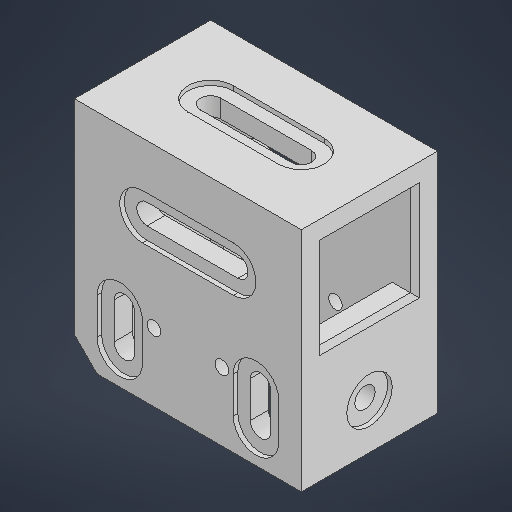
# Autodesk Inventor part: Part1
Saved by Autodesk Inventor 2025.1 (Build 291241000, 241)
## iProperties
Created: 2025-03-06
Part Number: Part1
Material: Generic
Document SubType Name: Modeling
Designer: jerem
Density: 1 g/cm^3
Appearance: Default
Author: jerem
Autodesk Inventor part; units mm, degrees
ref_plane "YZ Plane" through (0, 0, 0) normal (1, 0, 0) x (0, 1, 0)
ref_plane "XZ Plane" through (0, 0, 0) normal (0, 1, 0) x (-1, 0, 0)
ref_plane "XY Plane" through (0, 0, 0) normal (0, 0, 1) x (1, 0, 0)
sketch "Sketch1" plane through (0, 0, 0) normal (1, 0, 0) x (0, 1, 0)
  line L0 (-10, -10) -> (10, -10)
  line L1 (10, -10) -> (10, 10)
  line L2 (10, 10) -> (-10, 10)
  line L3 (-10, 10) -> (-10, -10)
  line L4 (-10, -10) -> (10, 10) construction
  line L5 (10, -10) -> (-10, 10) construction
  line L6 (-15, 15) -> (15, 15)
  line L7 (15, 15) -> (15, -15)
  line L8 (15, -15) -> (-15, -15)
  line L9 (-15, -15) -> (-15, 15)
  point P0 (0, 0)
  dimension "d0" = 20
  dimension "d1" = 20
  dimension "d2" = 5
  constraints: 20 end point, 4 parallel, 2 midpoint, 2 perpendicular, 1 horizontal, 3 other
  measures "d0" distance of L2.end L1.end
  measures "d1" distance of L1.end L0.end
  measures "d2" distance between parallel lines of L2 L6
extrude "Extrusion1" add sketch "Sketch1" along normal blind 40
sketch "Sketch2" plane through (0, 15, 15) normal (0, 1, 0) x (1, 0, 0)
  line L0 (0, 30) -> (0, 0) projected
  line L1 (0, 0) -> (40, 0) projected
  line L2 (40, 30) -> (40, 0) projected
  line L3 (0, 30) -> (40, 30) projected
  line L4 (0, 15) -> (10, 15) construction
  arc A0 (10, 17.25) -> (10, 12.75) centre (10, 15) ccw
  arc A1 (30, 12.75) -> (30, 17.25) centre (30, 15) ccw
  line L5 (10, 17.25) -> (30, 17.25)
  line L6 (30, 12.75) -> (10, 12.75)
  line L7 (20, 17.25) -> (20, 30) construction
  line L8 (30, 20) -> (10, 20)
  arc A2 (10, 20) -> (10, 10) centre (10, 15) ccw
  line L9 (10, 10) -> (30, 10)
  arc A3 (30, 10) -> (30, 20) centre (30, 15) ccw
  dimension "d5" = 4.5
  dimension "d7" = 20
  dimension "d8" = 10
  constraints: 12 end point, 8 point on circle, 4 centre point, 4 tangent, 2 midpoint, 2 perpendicular, 1 coincident, 1 equal radius, 1 horizontal, 3 other
  measures "d5" diameter of A0
  measures "d7" distance of A1.centre L4.end
  measures "d8" distance of L9.start L8.end
extrude "Extrusion2" cut sketch "Sketch2" against normal up to surface (5 mm away) contours L5 A1 L6 A0
extrude "Extrusion3" cut sketch "Sketch2" against normal blind 1 contours A3 L9 A2 L8
pattern_circular "Circular Pattern1" count 3 over 180 about axis through (-10, 0, 0) along (-1, 0, 0) of "Extrusion2", "Extrusion3" both ways yes
sketch "Sketch3" plane through (0, -15, -15) normal (0, -1, 0) x (1, 0, 0)
  line L0 (0, 30) -> (0, 0) projected
  line L1 (0, 0) -> (40, 0) projected
  line L2 (40, 30) -> (40, 0) projected
  line L3 (0, 30) -> (40, 30) projected
  line L4 (0, 15) -> (20, 15) construction
  line L5 (20, 30) -> (20, 15) construction
  line L6 (40, 5) -> (0, 5)
  line L7 (0, 5) -> (0, 25)
  line L8 (0, 25) -> (40, 25)
  line L9 (40, 25) -> (40, 5)
  line L10 (40, 5) -> (0, 25) construction
  line L11 (0, 5) -> (40, 25) construction
  line L12 (45, 30) -> (-5, 30)
  line L13 (-5, 30) -> (-5, 0)
  line L14 (-5, 0) -> (45, 0)
  line L15 (45, 0) -> (45, 30)
  point P0 (0, 5)
  point P1 (0, 25)
  point P2 (0, 30)
  dimension "d16" = 40
  dimension "d17" = 20
  dimension "d18" = 5
  constraints: 24 end point, 4 parallel, 3 midpoint, 2 horizontal, 2 perpendicular, 1 vertical, 3 other
  measures "d16" distance of L7.end L8.end
  measures "d17" distance of L6.end L7.end
  measures "d18" distance between parallel lines of L8 L12
extrude "Extrusion4" add sketch "Sketch3" along normal blind 20 contours L3 L2 L8 L0 | L0 L14 L13 L12 | L12 L15 L14 L2 | L6 L2 L1 L0
extrude "Extrusion5" cut sketch "Sketch3" against normal up to surface (5 mm away) contours L8 L2 L6 L0
sketch "Sketch4" plane through (45, -15, 15) normal (1, 0, 0) x (0, 0, -1)
  line L0 (0, 0) -> (0, -20) projected
  line L1 (30, -20) -> (0, -20) projected
  line L2 (30, 0) -> (30, -20) projected
  line L3 (30, 0) -> (0, 0) projected
  line L4 (15, 0) -> (15, -10) construction
  circle A0 centre (15, -10) radius 2.25
  circle A1 centre (15, -10) radius 5
  point P0 (15, 15)
  dimension "d23" = 10
  dimension "d24" = 4.5
  dimension "d25" = 10
  constraints: 2 centre point, 2 coincident, 2 end point, 1 midpoint, 1 vertical
  measures "d23" distance of L4.start L4.end
  measures "d24" diameter of A0
  measures "d25" diameter of A1
extrude "Extrusion6" cut sketch "Sketch4" against normal up to surface (5 mm away) contours A0
extrude "Extrusion11" cut sketch "Sketch4" against normal blind 1 contours A1
extrude "Extrusion7" add sketch "Sketch1" against normal up to surface (5 mm away)
extrude "Extrusion8" add sketch "Sketch1" along normal up to surface (5 mm away) from surface at 40
sketch "Sketch5" plane through (45, 15, -15) normal (0, 0, -1) x (-1, 0, 0)
  line L0 (50, 0) -> (0, 0) projected
  line L1 (0, 0) -> (0, -50) projected
  line L2 (50, -50) -> (0, -50) projected
  line L3 (15, -10) -> (35, -10) projected
  arc A0 (35, -20) -> (35, -10) centre (35, -15) ccw projected
  line L4 (35, -20) -> (15, -20) projected
  arc A1 (15, -10) -> (15, -20) centre (15, -15) ccw projected
  line L5 (0, -35) -> (10, -35) construction
  arc A2 (12.25, -35) -> (7.75, -35) centre (10, -35) ccw
  line L6 (10, -35) -> (10, -43) construction
  arc A3 (7.75, -43) -> (12.25, -43) centre (10, -43) ccw
  line L7 (12.25, -35) -> (12.25, -43)
  line L8 (7.75, -43) -> (7.75, -35)
  line L9 (5, -35) -> (5, -43)
  arc A4 (5, -43) -> (15, -43) centre (10, -43) ccw
  line L10 (15, -43) -> (15, -35)
  arc A5 (15, -35) -> (5, -35) centre (10, -35) ccw
  line L11 (25, -50) -> (25, -20) construction
  arc A6 (42.25, -35) -> (37.75, -35) centre (40, -35) ccw
  arc A7 (37.75, -43) -> (42.25, -43) centre (40, -43) ccw
  line L12 (37.75, -35) -> (37.75, -43)
  line L13 (42.25, -43) -> (42.25, -35)
  line L14 (45, -35) -> (45, -43)
  arc A8 (35, -43) -> (45, -43) centre (40, -43) ccw
  line L15 (35, -43) -> (35, -35)
  arc A9 (45, -35) -> (35, -35) centre (40, -35) ccw
  line L16 (50, -50) -> (50, 0) projected
  point P0 (45, -15)
  point P1 (0, -25)
  dimension "d35" = 10
  dimension "d37" = 4.5
  dimension "d38" = 10
  dimension "d39" = 8
  dimension "d40" = 10
  constraints: 22 end point, 16 point on circle, 10 symmetric about line, 8 centre point, 3 tangent, 2 coincident, 2 midpoint, 2 parallel, 2 vertical, 1 equal radius, 1 perpendicular, 1 point on line, 7 other
  measures "d35" distance of L5.start L5.end
  measures "d37" diameter of A2
  measures "d38" distance from line of point (0, -25) L5
  measures "d39" distance of L6.start L6.end
  measures "d40" distance of L10.end L9.start
extrude "Extrusion9" cut sketch "Sketch5" against normal up to surface (5 mm away) contours L7 A3 L8 A2 | L13 A7 L12 A6
extrude "Extrusion10" cut sketch "Sketch5" against normal blind 1 contours A5 L10 A4 L9 | L14 A8 L15 A9
mirror "Mirror1" about plane through (0, 0, 0) normal (0, 0, 1) of "Extrusion9", "Extrusion10"
chamfer "Chamfer2" distance 1 angle 45 11 edges at (45, 0, 10) (45, 10, 0) (45, 0, -10) (45, -10, 0) (-5, 0, 10) (-5, 10, 0) (-5, 0, -10) (-5, -10, 0) (20, -35, -10) (20, -35, 10) (40, -35, 0)
sketch "Sketch6" plane through (-5, 15, 15) normal (0, 0, 1) x (1, 0, 0)
  line L0 (35, -43) -> (35, -35) projected
  arc A0 (45, -35) -> (35, -35) centre (40, -35) ccw projected
  line L1 (45, -35) -> (45, -43) projected
  arc A1 (15, -35) -> (5, -35) centre (10, -35) ccw projected
  line L2 (15, -35) -> (15, -43) projected
  arc A2 (5, -43) -> (15, -43) centre (10, -43) ccw projected
  line L3 (5, -43) -> (5, -35) projected
  line L4 (50, -50) -> (0, -50) projected
  line L5 (50, 0) -> (50, -50) projected
  line L6 (0, 0) -> (50, 0) projected
  line L7 (35, -20) -> (15, -20) projected
  arc A3 (15, -10) -> (15, -20) centre (15, -15) ccw projected
  line L8 (15, -10) -> (35, -10) projected
  arc A4 (35, -20) -> (35, -10) centre (35, -15) ccw projected
  line L9 (25, -50) -> (25, -35) construction
  line L10 (17.5, -35) -> (32.5, -35) construction
  circle A5 centre (17.5, -35) radius 1.5
  circle A6 centre (32.5, -35) radius 1.5
  line L11 (25, -20) -> (25, -35) construction
  arc A7 (35, -43) -> (45, -43) centre (40, -43) ccw projected
  line L12 (0, 0) -> (0, -50) projected
  point P0 (5, -15)
  dimension "d50" = 3
  dimension "d51" = 15
  dimension "d52" = 15
  constraints: 6 end point, 4 midpoint, 2 centre point, 2 coincident, 2 vertical, 1 equal radius, 1 horizontal, 1 point on line
  measures "d50" diameter of A5
  measures "d51" distance of L10.start L10.end
  measures "d52" distance between parallel lines of L4 L10
extrude "Extrusion12" cut sketch "Sketch6" against normal through all contours A5 | A6
chamfer "Chamfer3" distance 5 angle 45 1 edges at (-5, -35, 0)
equation "\"d2\" = thickness"
equation "\"d18\" = thickness"
equation "\"thickness\" = 5"
body "Solid1"
